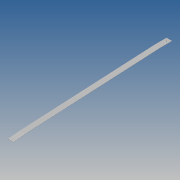
# Autodesk Inventor part: 2p6fs1
Saved by Autodesk Inventor 2014 SP1 (Build 180222100, 222)
## iProperties
Company: HERA Project
Created: 2013-12-11
Part Number: 2p6fs1
Material: Steel
Document SubType Name: Sheet Metal
Designer: David DeBoer
Mass: 925.881 g
Surface Area: 993.091 cm^2
Volume: 117.947 cm^3
Density: 7.85 g/cm^3
Description: inner furring strip
Appearance: Steel
Sheet Metal Rule: Default_mm
Author: David DeBoer
Autodesk Inventor part; units mm, degrees
ref_plane "YZ Plane" through (0, 0, 0) normal (1, 0, 0) x (0, 1, 0)
ref_plane "XZ Plane" through (0, 0, 0) normal (0, 1, 0) x (-1, 0, 0)
ref_plane "XY Plane" through (0, 0, 0) normal (0, 0, 1) x (1, 0, 0)
sketch "Sketch1" plane through (0, 0, 0) normal (0, 0, 1) x (1, 0, 0)
  line L0 (0, 0) -> (38.1, 0)
  line L1 (38.1, 0) -> (38.1, 1)
  line L2 (38.1, 1) -> (0, 1)
  line L3 (0, 1) -> (0, 0)
  dimension "d0" = 38.1
  dimension "d1" = 1
  constraints: 8 end point, 2 parallel, 1 horizontal, 1 perpendicular
  measures "d0" distance of L0.start L0.end
  measures "d1" distance of L2.end L0.start
extrude "Extrusion1" add sketch "Sketch1" along normal blind 1095
sketch "Sketch2" plane through (0, 1, 0) normal (0, 1, 0) x (1, 0, 0)
  line L0 (38.1, 0) -> (0, 0) projected
  circle A0 centre (19.05, -20) radius 2.2451
  dimension "d4" = 20
  constraints: 1 centre point
  measures "d4" distance from line of A0.centre L0
hole "Hole1" at (19.05, 1, 20) direction (0, -1, 0) diameter 5 end through all
sketch "Sketch3" plane through (0, 1, 0) normal (0, 1, 0) x (1, 0, 0)
  line L0 (38.1, -1095) -> (0, -1095) projected
  circle A0 centre (19.05, -1075) radius 2.2451
  dimension "d12" = 20
  constraints: 1 centre point
  measures "d12" distance from line of L0 A0.centre
hole "Hole2" at (19.05, 1, 1075) direction (0, -1, 0) diameter 5 end through all
sketch "Sketch6" plane through (0, 0, 0) normal (0, -1, 0) x (1, 0, 0)
  circle A0 centre (19.05, 20) radius 2.5 projected
  line L0 (38.1, 0) -> (38.1, 1095) projected
  line L1 (0, 0) -> (0, 1095) projected
  line L2 (0, 80) -> (38.1, 80) construction
  line L3 (0, 80) -> (38.1, 80)
  line L4 (0, 80) -> (60.428, 80) construction
  dimension "d29" = 60
  dimension "d30" = 0
  constraints: 6 end point, 3 point on line, 1 horizontal, 1 perpendicular
  measures "d29" distance from line of L2 A0.centre
  measures "d30" distance between parallel lines of L4 L3
fold "Fold2" angle 3 bend radius 1 thickness 1 k factor 0.44 line from (0, 0, 80) to (38.1, 0, 80) line at bend centre moving side (0, 0, 1) folds toward (0, -1, 0)
sketch "Sketch7" plane through (0, -0.0014, 80.0146) normal (0, -0.9986295, -0.052336) x (1, 0, 0)
  line L0 (38.1, 0) -> (38.1, 1014.9623) projected
  line L1 (0, 0) -> (0, 1014.9623) projected
  line L2 (0, 934.9623) -> (38.1, 934.9623) construction
  line L3 (0, 934.9623) -> (38.1, 934.9623)
  line L4 (0, 934.9623) -> (38.1, 934.9623) construction
  circle A0 centre (19.05, 994.9623) radius 2.5 projected
  point P0 (0, -79.9051)
  dimension "d37" = 0
  dimension "d44" = 60
  constraints: 6 end point, 3 point on line, 1 horizontal, 1 perpendicular
  measures "d37" distance between parallel lines of L3 L4
  measures "d44" distance from line of L2 A0.centre
fold "Fold3" angle 3 bend radius 1 thickness 1 k factor 0.44 line from (0, -48.9335, 1013.6956) to (38.1, -48.9335, 1013.6956) line at bend centre moving side (0, -0.052336, 0.9986295) folds toward (0, -0.9986295, -0.052336)
sketch "Sketch8" plane through (0, 0.9973, 80.067) normal (0, 0.9986295, 0.052336) x (1, 0, 0)
  line L0 (38.1, 0) -> (38.1, -934.9246) projected
  line L1 (0, 0) -> (0, -934.9246) projected
  line L2 (0, -467.4623) -> (38.1, -467.4623)
  circle A0 centre (19.05, -367.4623) radius 9.5512
  circle A1 centre (19.05, -567.4623) radius 9.5512
  point P0 (0, 79.9051)
  dimension "d45" = 100
  constraints: 2 centre point, 2 end point, 2 midpoint, 1 symmetric about line, 1 other
  measures "d45" distance from line of A0.centre L2
hole "Hole3" at (19.05, -28.7014, 646.7516) at (19.05, -18.2342, 447.0257) direction (0, -0.9986295, -0.052336) diameter 1 end through all
equation "\"d1\" = Thickness"
equation "\"d31\" = BendReliefWidth"
equation "\"d32\" = BendReliefDepth"
equation "\"d33\" = MinimumRemnant"
equation "\"d34\" = BendRadius"
equation "\"d36\" = BendRadius"
equation "\"d38\" = BendReliefWidth"
equation "\"d39\" = BendReliefDepth"
equation "\"d40\" = MinimumRemnant"
equation "\"d41\" = BendRadius"
equation "\"d43\" = BendRadius"
equation "\"d51\" = Thickness"
equation "\"BendRadius\" = Thickness"
equation "\"BendReliefWidth\" = Thickness"
equation "\"BendReliefDepth\" = 0.5 * Thickness"
equation "\"CornerReliefSize\" = 4 * Thickness"
equation "\"MinimumRemnant\" = 2 * Thickness"
equation "\"TransitionRadius\" = BendRadius"
equation "\"JacobiRadiusSize\" = BendRadius"
equation "\"GapSize\" = Thickness"
equation "\"Thickness\" = 1"
body "Solid1"
